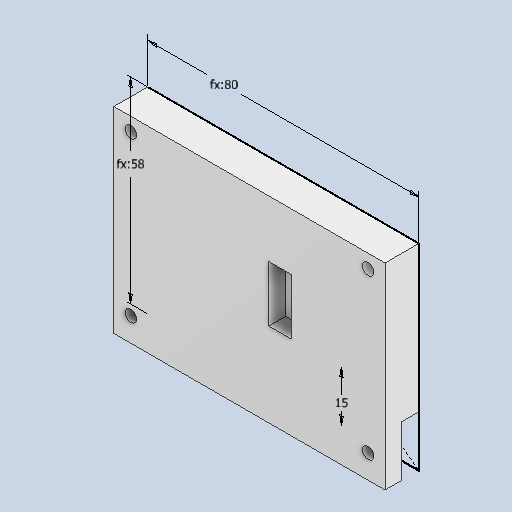
# Autodesk Inventor part: Sensor_Box_Deckel
Saved by Autodesk Inventor 2024 (Build 280153000, 153)
## iProperties
Created: 2022-10-05
Part Number: Sensor_Box_Deckel
Material: PBT-Kunststoff
Document SubType Name: Modeling
Designer: alexw
Density: 1.31 g/cm^3
Appearance: Glatt - Weiß
Mass: 59.9032 g
Surface Area: 133.978 cm^2
Volume: 45.7276 cm^3
Author: alexw
Autodesk Inventor part; units mm, degrees
ref_plane "YZ Plane" through (0, 0, 0) normal (1, 0, 0) x (0, 1, 0)
ref_plane "XZ Plane" through (0, 0, 0) normal (0, 1, 0) x (-1, 0, 0)
ref_plane "XY Plane" through (0, 0, 0) normal (0, 0, 1) x (1, 0, 0)
sketch "Skizze1" plane through (0, 0, 0) normal (0, 0, 1) x (1, 0, 0)
  line L0 (-40, 29) -> (40, 29)
  line L1 (40, 29) -> (40, -29)
  line L2 (40, -29) -> (-40, -29)
  line L3 (-40, -29) -> (-40, 29)
  line L4 (-40, 29) -> (40, -29) construction
  line L5 (40, 29) -> (-40, -29) construction
  line L6 (-40, -14) -> (40, -14)
  point P0 (0, 0)
  dimension "d0" = 58
  dimension "d1" = 80
  dimension "d4" = 15
  constraints: 14 end point, 2 midpoint, 2 parallel, 2 perpendicular, 2 point on line, 1 horizontal
  measures "d0" distance of L2.end L0.start
  measures "d1" distance of L0.start L0.end
  measures "d4" distance between parallel lines of L6 L2
extrude "Extrusion1" add sketch "Skizze1" along normal blind 10
extrude "Extrusion2" cut sketch "Skizze1" along normal blind 5 contours L6 L1 L2 L3
sketch "Skizze2" plane through (0, 0, 0) normal (0, 0, -1) x (-1, 0, 0)
  line L0 (35, -22) -> (-35, -22) construction
  line L1 (-40, -14) -> (40, -14) projected
  line L2 (0, -14) -> (0, -22) construction
  line L3 (40, -14) -> (40, -29) projected
  line L4 (35, 25) -> (-35, 25) construction
  line L5 (-40, 29) -> (40, 29) projected
  point P0 (0, 0)
  point P1 (0, 25)
  dimension "d7" = 8
  dimension "d8" = 5
  dimension "d16" = 70
  dimension "d17" = 4
  constraints: 6 end point, 4 coincident, 3 midpoint, 2 horizontal, 1 point on line, 1 vertical
  measures "d7" distance between parallel lines of L1 L0
  measures "d8" distance from line of L3 L0.start
  measures "d16" distance of L4.start L4.end
  measures "d17" distance between parallel lines of L5 L4
hole "Bohrung1" at (-35, -22, 0) at (35, -22, 0) at (-35, 25, 0) at (35, 25, 0) direction (0, 0, 1) diameter 3.4 end through all clearance for "Inbusschraube DIN EN ISO 4762" size "M3" standard "DIN"
sketch "Sketch3" plane through (0, 0, 0) normal (0, 0, -1) x (-1, 0, 0)
  line L0 (-30.5, 21) -> (-30.5, -14) projected
  line L1 (-4, 21) -> (-30.5, 21) projected
  line L2 (-4, -14) -> (-4, 21) projected
  line L3 (-4, -14) -> (-30.5, -14)
  point P0 (0, 0)
  constraints: 2 end point, 1 horizontal
extrude "Extrusion3" cut sketch "Sketch3" against normal up to surface (5 mm away)
sketch "Sketch4" plane through (0, 0, 5) normal (0, 0, -1) x (-1, 0, 0)
  line L0 (-12.32, -4.25) -> (-5.72, -4.25)
  line L1 (-5.72, -4.25) -> (-5.72, 12.25)
  line L2 (-5.72, 12.25) -> (-12.32, 12.25)
  line L3 (-12.32, 12.25) -> (-12.32, -4.25)
  line L4 (-10.2773, -2.3373) -> (-7.7627, -2.3373) projected
  line L5 (-7.7627, 10.3373) -> (-10.2773, 10.3373) projected
  line L6 (-10.2773, -2.3373) -> (-7.7627, -2.3373)
  line L7 (-7.7627, -2.3373) -> (-7.7627, 10.3373)
  line L8 (-7.7627, 10.3373) -> (-10.2773, 10.3373)
  line L9 (-10.2773, 10.3373) -> (-10.2773, -2.3373)
  line L10 (-10.2773, 4) -> (-12.32, 4) construction
  line L11 (-9.02, -2.3373) -> (-9.02, -4.25) construction
  point P0 (0, 0)
  dimension "d20" = 6.6
  dimension "d21" = 16.5
  constraints: 20 end point, 4 midpoint, 4 parallel, 3 horizontal, 2 perpendicular, 1 vertical
  measures "d20" distance of L1.end L2.end
  measures "d21" distance of L2.end L0.start
extrude "Extrusion4" cut sketch "Sketch4" against normal through all contours L3 L2 L1 L0 | L9 L5 L7 L4
equation "\"d0\" = SensorBox_Width"
equation "\"d1\" = SensorBox_Length"
equation "\"SensorBox_Width\" = 58"
equation "\"SensorBox_Length\" = 80"
